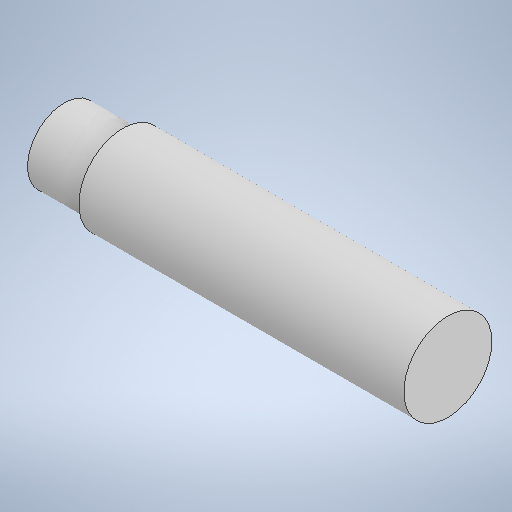
# Autodesk Inventor part: welle 30
Saved by Autodesk Inventor 2025.1 (Build 291241000, 241)
## iProperties
Created: 2024-09-13
Part Number: welle 30
Material: Generisch
Document SubType Name: Modeling
Designer: ffogue
Density: 1 g/cm^3
Appearance: Vorgabe
Author: ffogue
Autodesk Inventor part; units mm, degrees
ref_plane "YZ Plane" through (0, 0, 0) normal (1, 0, 0) x (0, 1, 0)
ref_plane "XZ Plane" through (0, 0, 0) normal (0, 1, 0) x (-1, 0, 0)
ref_plane "XY Plane" through (0, 0, 0) normal (0, 0, 1) x (1, 0, 0)
sketch "Sketch1" plane through (0, 0, 0) normal (0, 0, 1) x (1, 0, 0)
  line L0 (0, 0) -> (0, 2.5)
  line L1 (0, 2.5) -> (4, 2.5)
  line L2 (4, 2.5) -> (4, 3)
  line L3 (4, 3) -> (26.16, 3)
  line L4 (26.16, 3) -> (26.16, 0)
  line L5 (26.16, 0) -> (0, 0)
  dimension "d0" = 4
  dimension "d2" = 5
  dimension "d3" = 6
  dimension "d6" = 22.16
  constraints: 12 end point, 4 perpendicular, 1 parallel, 1 vertical
  measures "d0" distance of L0.end L1.end
  measures "d2" diameter of L1 L5
  measures "d3" diameter of L3 L5
  measures "d6" distance of L2.end L3.end
revolve "Revolution1" add sketch "Sketch1" angle 360 about axis through (26.16, 0, 0) along (-1, 0, 0)
sketch "Sketch3" plane through (26.16, 0, 0) normal (1, 0, 0) x (0, 0, -1)
  circle A0 centre (0, 0) radius 3 projected
body "Solid1"
